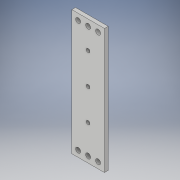
# Autodesk Inventor part: 000.405 - Рычаг
Saved by Autodesk Inventor 2019 (Build 230136000, 136)
## iProperties
Created: 2020-02-28
Part Number: 000.405 - Рычаг
Material: Типовые
Document SubType Name: Modeling
Designer: Петров Иван
Density: 1 g/cm^3
Appearance: По умолчанию
Author: Петров Иван
Autodesk Inventor part; units mm, degrees
ref_plane "YZ Plane" through (0, 0, 0) normal (1, 0, 0) x (0, 1, 0)
ref_plane "XZ Plane" through (0, 0, 0) normal (0, 1, 0) x (-1, 0, 0)
ref_plane "XY Plane" through (0, 0, 0) normal (0, 0, 1) x (1, 0, 0)
sketch "Эскиз1" plane through (0, 0, 0) normal (0, 0, 1) x (1, 0, 0)
  line L0 (0, 0) -> (26.2, 0)
  line L1 (26.2, 0) -> (26.2, 100)
  line L2 (26.2, 100) -> (0, 100)
  line L3 (0, 100) -> (0, 0)
  dimension "d0" = 26.2
  dimension "d1" = 100
  constraints: 8 end point, 2 parallel, 1 horizontal, 1 perpendicular
  measures "d0" distance of L1.end L2.end
  measures "d1" distance of L0.end L1.end
extrude "Выдавливание1" add sketch "Эскиз1" along normal blind 3
sketch "Эскиз2" plane through (0, 0, 3) normal (0, 0, 1) x (1, 0, 0)
  line L0 (0, 0) -> (26.2, 0) projected
  line L1 (13.1, 0) -> (13.1, 5)
  circle A0 centre (13.1, 5) radius 2
  dimension "d4" = 5
  dimension "d5" = 4
  constraints: 2 end point, 1 centre point, 1 coincident, 1 midpoint, 1 vertical
  measures "d4" distance of L1.start L1.end
  measures "d5" diameter of A0
extrude "Выдавливание2" cut sketch "Эскиз2" against normal blind 3
pattern_linear "Прямоуг.массив1" count 3 spacing 8 along (1, 0, 0) of "Выдавливание2" first direction both ways yes
sketch "Эскиз3" plane through (0, 0, 3) normal (0, 0, 1) x (1, 0, 0)
  line L0 (26.2, 0) -> (26.2, 100) projected
  line L1 (26.2, 28.1365) -> (26.2, 15.0365)
  line L2 (26.2, 28.1365) -> (13.1, 28.1365)
  circle A0 centre (13.1, 28.1365) radius 1.5
  point P0 (0, 0)
  dimension "d12" = 13.1
  dimension "d13" = 3
  constraints: 4 end point, 2 point on line, 1 centre point, 1 coincident, 1 horizontal
  measures "d12" distance of L1.start L2.end
  measures "d13" diameter of A0
extrude "Выдавливание3" cut sketch "Эскиз3" against normal blind 3
pattern_linear "Прямоуг.массив2" count 3 spacing 25 along (0, 1, 0) of "Выдавливание3"
ref_plane "РабПлоскость1" through (26.2, 50, 3) normal (0, 1, 0) x (1, 0, 0)
mirror "Зеркальное отражение1" about plane through (26.2, 50, 3) normal (0, 1, 0) of "Выдавливание2", "Прямоуг.массив1"
